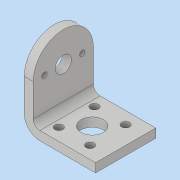
# Autodesk Inventor part: 联轴器
Saved by Autodesk Inventor 2019 (Build 230136000, 136)
## iProperties
Created: 2020-11-01
Part Number: 联轴器
Material: Generic
Document SubType Name: Modeling
Designer: Wang Hua
Density: 1 g/cm^3
Appearance: Default
Author: Wang Hua
Autodesk Inventor part; units mm, degrees
ref_plane "YZ Plane" through (0, 0, 0) normal (1, 0, 0) x (0, 1, 0)
ref_plane "XZ Plane" through (0, 0, 0) normal (0, 1, 0) x (-1, 0, 0)
ref_plane "XY Plane" through (0, 0, 0) normal (0, 0, 1) x (1, 0, 0)
sketch "草图1" plane through (0, 0, 0) normal (0, 0, 1) x (1, 0, 0)
  line L0 (-17.146, 12.8249) -> (-13.146, 12.8249)
  line L1 (-13.146, 12.8249) -> (-13.146, -15.1751)
  line L2 (-17.146, -15.1751) -> (-17.146, 12.8249)
  arc A0 (-13.146, -15.1751) -> (-10.146, -18.1751) centre (-10.146, -15.1751) ccw
  line L3 (-10.146, -18.1751) -> (-10.146, -15.1751) construction
  arc A1 (-17.146, -15.1751) -> (-10.146, -22.1751) centre (-10.146, -15.1751) ccw
  line L4 (-10.146, -18.1751) -> (14.854, -18.1751)
  line L5 (-10.146, -22.1751) -> (14.854, -22.1751)
  line L6 (14.854, -18.1751) -> (14.854, -22.1751)
  point P0 (0, 0)
  dimension "d0" = 4
  dimension "d1" = 28
  dimension "d2" = 28
  dimension "d3" = 3
  dimension "d4" = 25
  dimension "d5" = 25
  constraints: 14 end point, 4 point on circle, 3 horizontal, 2 centre point, 2 parallel, 1 coincident, 1 perpendicular, 1 point on line
  measures "d0" distance of L0.start L0.end
  measures "d1" distance of L2.start L0.start
  measures "d2" distance of L0.end L1.end
  measures "d3" radius of A0
  measures "d4" distance of L3.start L4.end
  measures "d5" distance of L5.start L5.end
extrude "拉伸1" add sketch "草图1" along normal blind 27
sketch "草图2" plane through (-17.146, -15.1751, 0) normal (-1, 0, 0) x (0, 0, 1)
  line L0 (0, 28) -> (0, 0) construction
  line L1 (27, 0) -> (27, -3) construction
  line L2 (0, 28) -> (27, 28) construction
  line L3 (27, 28) -> (27, 0) construction
  line L4 (27, 0) -> (0, 0) construction
  line L5 (0, 0) -> (0, 28) construction
  line L6 (0, 14.5) -> (27, 14.5) construction
  line L7 (27, 0) -> (27, 28) construction
  point P0 (0, 15.1751)
  dimension "d8" = 13.5
  constraints: 10 end point, 3 parallel, 2 point on line, 1 horizontal, 1 perpendicular
  measures "d8" distance between parallel lines of L6 L2
sketch "草图3" plane through (-13.146, -15.1751, 0) normal (1, 0, 0) x (0, 0, -1)
  line L0 (-27, 0) -> (-27, 28) construction
  line L1 (0, 0) -> (0, -3) construction
  line L2 (-27, 28) -> (0, 28) construction
  line L3 (0, 28) -> (0, 0) construction
  line L4 (0, 0) -> (-27, 0) construction
  line L5 (-27, 0) -> (-27, 28) construction
  line L6 (-27, 14.5) -> (0, 14.5) construction
  line L7 (0, 28) -> (-27, 28) construction
  arc A0 (0, 14.5) -> (-27, 14.5) centre (-13.5, 14.5) ccw
  line L8 (-27, 14.5) -> (-27, 28)
  line L9 (-13.5, 28) -> (-27, 28)
  line L10 (-13.5, 28) -> (0, 28)
  line L11 (0, 28) -> (0, 0) projected
  line L12 (0, 14.5) -> (0, 28)
  circle A1 centre (-13.5, 14.5) radius 3.6
  circle A2 centre (-5, 14.5) radius 1.23
  line L13 (-13.5, 14.5) -> (-13.5, 0) construction
  circle A3 centre (-22, 14.5) radius 1.23
  point P0 (0, 15.1751)
  dimension "d9" = 13.5
  dimension "d12" = 7.2
  dimension "d13" = 2.46
  dimension "d14" = 17
  constraints: 20 end point, 4 centre point, 4 collinear, 3 midpoint, 3 parallel, 3 point on circle, 3 point on line, 2 tangent, 1 coincident, 1 horizontal, 1 perpendicular, 1 symmetric about line, 1 other
  measures "d9" distance between parallel lines of L2 L6
  measures "d12" diameter of A1
  measures "d13" diameter of A2
  measures "d14" distance of A2.centre A3.centre
extrude "拉伸2" cut sketch "草图3" against normal through all contours A0 L8 L9 | A0 L10 L11
extrude "拉伸3" cut sketch "草图3" against normal through all contours A1 | A2 | A3
sketch "草图4" plane through (-10.146, -18.1751, 0) normal (0, 1, 0) x (1, 0, 0)
  point P0 (10.146, 0)
sketch "草图5" plane through (-10.146, -18.1751, 0) normal (0, 1, 0) x (1, 0, 0)
  circle A0 centre (10, -13.5) radius 5
  line L0 (25, 0) -> (0, 0) projected
  line L1 (25, 0) -> (25, -27) projected
  line L2 (10, -13.5) -> (10, -3.684) construction
  line L3 (10, -13.5) -> (-1.3209, -13.5) construction
  point P0 (10.146, 0)
  point P1 (3, -5.5)
  point P2 (3, -21.5)
  point P3 (17, -5.5)
  point P4 (17, -21.5)
  dimension "d17" = 10
  dimension "d18" = 13.5
  dimension "d19" = 15
  dimension "d20" = 16
  dimension "d21" = 14
  dimension "d22" = 7
  dimension "d23" = 7
  constraints: 4 end point, 2 symmetric about line, 1 centre point, 1 horizontal, 1 vertical
  measures "d17" diameter of A0
  measures "d18" distance from line of L2.start L0
  measures "d19" distance from line of L1 L2.start
  measures "d20" distance of point (3, -21.5) point (3, -5.5)
  measures "d21" distance of point (17, -5.5) point (3, -5.5)
  measures "d22" distance from line of L2 point (3, -5.5)
  measures "d23" distance from line of L2 point (17, -21.5)
extrude "拉伸4" cut sketch "草图5" against normal through all
hole "孔1" at (-7.146, -18.1751, 21.5) at (-7.146, -18.1751, 5.5) at (6.854, -18.1751, 5.5) at (6.854, -18.1751, 21.5) direction (0, -1, 0) diameter 3.6 end through all
